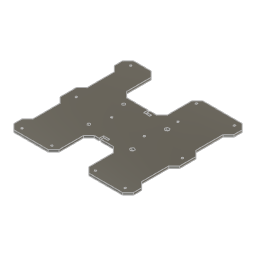
cr6_buildplate_carriage (Autodesk Fusion 360 design; units mm, degrees)
Autodesk Fusion 360 part; units mm, degrees
note: some values were not read from the file. Set by a fixed rule: the direction of a hole.
sketch "Sketch1" plane through (0, 0, 0) normal (0, 0, 1) x (1, 0, 0)
  line L0 (10, 0) -> (210, 0)
  line L1 (220, 10) -> (220, 210)
  line L2 (210, 220) -> (10, 220)
  line L3 (0, 210) -> (0, 10)
  line L4 (83, 0) -> (138, 0)
  line L5 (138, 0) -> (138, 55)
  line L6 (128, 65) -> (93, 65)
  line L7 (83, 55) -> (83, 0)
  line L8 (52.5, 220) -> (127.5, 220)
  line L9 (127.5, 220) -> (127.5, 165)
  line L10 (117.5, 155) -> (62.5, 155)
  line L11 (52.5, 165) -> (52.5, 220)
  line L12 (52.5, 165) -> (62.5, 155)
  line L13 (117.5, 155) -> (127.5, 165)
  line L14 (83, 55) -> (93, 65)
  line L15 (128, 65) -> (138, 55)
  line L16 (0, 25) -> (10, 25)
  line L17 (10, 25) -> (10, 95)
  line L18 (10, 95) -> (0, 95)
  line L19 (0, 95) -> (0, 25)
  line L20 (0, 125) -> (10, 125)
  line L21 (10, 125) -> (10, 195)
  line L22 (10, 195) -> (0, 195)
  line L23 (0, 195) -> (0, 125)
  line L24 (10, 220) -> (0, 210)
  line L25 (210, 220) -> (220, 210)
  line L26 (0, 10) -> (10, 0)
  line L27 (210, 0) -> (220, 10)
  line L28 (0, 95) -> (10, 85)
  line L29 (0, 125) -> (10, 135)
  line L30 (0, 195) -> (10, 185)
  line L31 (0, 25) -> (10, 35)
  line L32 (110, 0) -> (110, 220) construction
  line L33 (210, 195) -> (220, 195)
  line L34 (220, 195) -> (210, 185)
  line L35 (210, 125) -> (210, 195)
  line L36 (220, 125) -> (210, 135)
  line L37 (220, 125) -> (210, 125)
  line L38 (210, 95) -> (220, 95)
  line L39 (210, 25) -> (210, 95)
  line L40 (220, 95) -> (210, 85)
  line L41 (220, 25) -> (210, 25)
  line L42 (220, 25) -> (210, 35)
  line L43 (0, 110) -> (220, 110) construction
  line L44 (150, 142) -> (70, 142) construction
  line L45 (70, 142) -> (70, 78) construction
  line L46 (70, 78) -> (150, 78) construction
  line L47 (150, 78) -> (150, 142) construction
  line L48 (150, 142) -> (70, 78) construction
  line L49 (70, 142) -> (150, 78) construction
  line L50 (102, 65) -> (102, 73)
  line L51 (102, 73) -> (113, 73)
  line L52 (113, 73) -> (113, 70)
  line L53 (113, 70) -> (105, 70)
  line L54 (105, 70) -> (105, 65)
  line L55 (102, 155) -> (102, 147)
  line L56 (102, 147) -> (113, 147)
  line L57 (113, 150) -> (105, 150)
  line L58 (113, 147) -> (113, 150)
  line L59 (105, 150) -> (105, 155)
  line L60 (42.5, 220) -> (52.5, 210)
  line L61 (127.5, 210) -> (137.5, 220)
  line L62 (138, 10) -> (148, 0)
  line L63 (83, 10) -> (73, 0)
  point P0 (220, 0)
  point P1 (0, 220)
  point P2 (52.5, 155)
  point P3 (127.5, 155)
  point P4 (83, 65)
  point P5 (138, 65)
  point P6 (220, 220)
  point P7 (110, 110)
  point P8 (110, 110)
  dimension "d1" = 220
  dimension "d2" = 220
  dimension "d3" = 83
  dimension "d4" = 138
  dimension "d5" = 65
  dimension "d6" = 52.5
  dimension "d7" = 127.5
  dimension "d8" = 65
  dimension "d9" = 10
  dimension "d10" = 10
  dimension "d11" = 10
  dimension "d12" = 10
  dimension "d13" = 10
  dimension "d14" = 10
  dimension "d15" = 10
  dimension "d16" = 10
  dimension "d17" = 95
  dimension "d18" = 25
  dimension "d19" = 10
  dimension "d20" = 195
  dimension "d21" = 125
  dimension "d22" = 10
  dimension "d23" = 10
  dimension "d24" = 10
  dimension "d25" = 10
  dimension "d26" = 10
  dimension "d27" = 10
  dimension "d28" = 10
  dimension "d29" = 10
  dimension "d30" = 10
  dimension "d31" = 80
  dimension "d32" = 64
  dimension "d41" = 102
  dimension "d42" = 3
  dimension "d44" = 3
  dimension "d45" = 11
  dimension "d46" = 8
  dimension "d60" = 10
  dimension "d61" = 10
  dimension "d62" = 10
  dimension "d63" = 10
  constraint horizontal L0
  constraint vertical L1
  constraint horizontal L2
  constraint vertical L3
  constraint horizontal L4
  constraint vertical L5
  constraint horizontal L6
  constraint vertical L7
  constraint coincident L0 L4.start
  constraint horizontal L8
  constraint vertical L9
  constraint horizontal L10
  constraint vertical L11
  constraint coincident L2 L8.start
  constraint coincident L11 P2
  constraint coincident L10 P2
  constraint coincident L10 P3
  constraint coincident L9 P3
  constraint coincident L7 P4
  constraint coincident L6 P4
  constraint coincident L6 P5
  constraint coincident L5 P5
  constraint horizontal L16
  constraint vertical L17
  constraint horizontal L18
  constraint vertical L19
  constraint coincident L3 L16.start
  constraint horizontal L20
  constraint vertical L21
  constraint horizontal L22
  constraint vertical L23
  constraint coincident L3 L20.start
  constraint coincident P1 L2
  constraint coincident P1 L3
  constraint coincident L2 P6
  constraint coincident L1 P6
  constraint coincident origin L3
  constraint coincident origin L0
  constraint coincident P0 L0
  constraint coincident P0 L1
  constraint coincident L17 L28.end
  constraint coincident L21 L29.end
  constraint perpendicular L28 L29
  constraint coincident L21 L30.end
  constraint perpendicular L29 L30
  constraint coincident L17 L31.end
  constraint perpendicular L30 L31
  constraint midpoint L0 L32.start
  constraint midpoint L2 L32.end
  constraint symmetric L16.start L32 L41.start
  constraint symmetric L16.end L32 L39.start
  constraint symmetric L17.end L32 L38.start
  constraint symmetric L18.end L32 L38.end
  constraint symmetric L20.start L32 L36.start
  constraint symmetric L20.end L32 L35.start
  constraint symmetric L21.end L32 L33.start
  constraint symmetric L22.end L32 L33.end
  constraint symmetric L28.end L32 L40.end
  constraint symmetric L29.end L32 L36.end
  constraint symmetric L30.end L32 L34.end
  constraint symmetric L31.end L32 L42.end
  constraint midpoint L3 L43.start
  constraint midpoint L1 L43.end
  constraint midpoint L32 P8
  constraint horizontal L44
  constraint perpendicular L44 L45
  constraint parallel L44 L46
  constraint parallel L45 L47
  constraint coincident L48 P8
  constraint coincident L49 P8
  constraint coincident P8 P7
  constraint coincident L6 L50.start
  constraint perpendicular L6 L50
  constraint perpendicular L50 L51
  constraint perpendicular L51 L52
  constraint perpendicular L52 L53
  constraint coincident L6 L54.end
  constraint perpendicular L6 L54
  constraint symmetric L43 L50.start L55.start
  constraint symmetric L43 L50.end L55.end
  constraint symmetric L43 L51.end L56.end
  constraint symmetric L43 L52.end L57.start
  constraint symmetric L43 L53.end L57.end
  constraint symmetric L43 L54.end L59.end
  constraint coincident L2 L60.start
  constraint coincident L11 L60.end
  constraint perpendicular L24 L60
  constraint coincident L9 L61.start
  constraint coincident L2 L61.end
  constraint perpendicular L60 L61
  constraint coincident L5 L62.start
  constraint coincident L0 L62.end
  constraint perpendicular L61 L62
  constraint coincident L7 L63.start
  constraint coincident L0 L63.end
  constraint perpendicular L62 L63
  measures "d1" distance of origin P0
  measures "d2" distance of origin P1
  measures "d3" distance of L3 L7
  measures "d4" distance of L3 L5
  measures "d5" distance of L0 L6
  measures "d6" distance of L3 L11
  measures "d7" distance of L3 L9
  measures "d8" distance of L2 L10
  measures "d9" distance of L11.start P2
  measures "d10" distance of L10.end P2
  measures "d11" distance of L10.start P3
  measures "d12" distance of L9.end P3
  measures "d13" distance of L7.start P4
  measures "d14" distance of L6.end P4
  measures "d15" distance of L6.start P5
  measures "d16" distance of L5.end P5
  measures "d17" distance of L0 L18
  measures "d18" distance of L0 L16
  measures "d19" distance of L17 L19
  measures "d20" distance of L0 L22
  measures "d21" distance of L0 L20
  measures "d22" distance of L3 L21
  measures "d23" distance of P1 L2.end
  measures "d24" distance of P1 L3.start
  measures "d25" distance of L2.start P6
  measures "d26" distance of L1.end P6
  measures "d27" distance of origin L3.end
  measures "d28" distance of origin L0.start
  measures "d29" distance of P0 L0.end
  measures "d30" distance of P0 L1.start
  measures "d31" distance of L45.end L46.end
  measures "d32" distance of L44.end L45.end
  measures "d41" distance of L3 L50
  measures "d42" distance of L50 L54
  measures "d44" distance of L51 L53
  measures "d45" distance of L50 L52
  measures "d46" distance of L6 L51
  measures "d60" distance of L8.start L60.start
  measures "d61" distance of L8.end L61.end
  measures "d62" distance of L4.start L63.end
  measures "d63" horizontal distance of L62.start L62.end
extrude "Extrude1" add sketch "Sketch1" along normal blind 4 contours L0 L1 L2 L3 L5 L6 L7 L9 L10 L11 L12 L13 L14 L15 L16 L17 L18 L20 L21 L22 L24 L25 L26 L27 L33 L35 L37 L38 L39 L41 L50 L51 L52 L53 L54 L55 L56 L57 L58 L59 L60 L61 L62 L63 | L16 L17 L31 | L17 L18 L28 | L20 L21 L29 | L21 L22 L30 | L39 L41 L42 | L38 L39 L40 | L35 L36 L37 | L33 L34 L35
hole "Hole1" at (70, 142, 0) at (70, 78, 0) direction (0, 0, 1) diameter 5 end through all
hole "Hole2" at (150, 78, 0) at (150, 142, 0) direction (0, 0, 1) diameter 7.2 depth 4 tip angle 118
sketch "Sketch2" plane through (0, 0, 4) normal (0, 0, 1) x (-1, 0, 0)
  circle A0 centre (-150, -78) radius 3.6
  circle A1 centre (-150, -142) radius 3.6
  circle A2 centre (-70, -142) radius 2.5
  circle A3 centre (-70, -78) radius 2.5
  line L0 (-102, -155) -> (-62.5, -155)
  line L1 (-62.5, -155) -> (-52.5, -165)
  line L2 (-52.5, -165) -> (-52.5, -210)
  line L3 (-42.5, -220) -> (-10, -220)
  line L4 (-10, -220) -> (0, -210)
  line L5 (0, -210) -> (0, -195)
  line L6 (0, -195) -> (-10, -185)
  line L7 (-10, -185) -> (-10, -135)
  line L8 (-10, -135) -> (0, -125)
  line L9 (0, -125) -> (0, -95)
  line L10 (0, -95) -> (-10, -85)
  line L11 (-10, -85) -> (-10, -35)
  line L12 (-10, -35) -> (0, -25)
  line L13 (0, -25) -> (0, -10)
  line L14 (0, -10) -> (-10, 0)
  line L15 (-10, 0) -> (-73, 0)
  line L16 (-83, -10) -> (-83, -55)
  line L17 (-83, -55) -> (-93, -65)
  line L18 (-93, -65) -> (-102, -65)
  line L19 (-102, -65) -> (-102, -73)
  line L20 (-102, -73) -> (-113, -73)
  line L21 (-113, -73) -> (-113, -70)
  line L22 (-113, -70) -> (-105, -70)
  line L23 (-105, -70) -> (-105, -65)
  line L24 (-105, -65) -> (-128, -65)
  line L25 (-128, -65) -> (-138, -55)
  line L26 (-138, -55) -> (-138, -10)
  line L27 (-148, 0) -> (-210, 0)
  line L28 (-210, 0) -> (-220, -10)
  line L29 (-220, -10) -> (-220, -25)
  line L30 (-220, -25) -> (-210, -35)
  line L31 (-210, -35) -> (-210, -85)
  line L32 (-210, -85) -> (-220, -95)
  line L33 (-220, -95) -> (-220, -125)
  line L34 (-220, -125) -> (-210, -135)
  line L35 (-210, -135) -> (-210, -185)
  line L36 (-210, -185) -> (-220, -195)
  line L37 (-220, -195) -> (-220, -210)
  line L38 (-220, -210) -> (-210, -220)
  line L39 (-210, -220) -> (-137.5, -220)
  line L40 (-127.5, -210) -> (-127.5, -165)
  line L41 (-127.5, -165) -> (-117.5, -155)
  line L42 (-117.5, -155) -> (-105, -155)
  line L43 (-105, -155) -> (-105, -150)
  line L44 (-105, -150) -> (-113, -150)
  line L45 (-113, -150) -> (-113, -147)
  line L46 (-113, -147) -> (-102, -147)
  line L47 (-102, -147) -> (-102, -155)
  line L48 (0, -110) -> (-220, -110) construction
  line L49 (-10, 0) -> (-210, 0) construction
  line L50 (0, -10) -> (-220, -10) construction
  line L51 (0, -210) -> (-220, -210) construction
  line L52 (-138, -10) -> (-148, 0)
  line L53 (-137.5, -220) -> (-127.5, -210)
  line L54 (-52.5, -210) -> (-42.5, -220)
  line L55 (-73, 0) -> (-83, -10)
  point P0 (-15, -110)
  point P1 (-80, -110)
  point P2 (-140, -110)
  point P3 (-210, -110)
  point P4 (-15, -210)
  point P5 (-136, -210)
  point P6 (-206, -210)
  point P7 (-15, -10)
  point P8 (-70, -10)
  point P9 (-150, -10)
  point P10 (-205, -10)
  point P11 (-148, -164)
  dimension "d47" = 110
  dimension "d48" = 10
  dimension "d49" = 15
  dimension "d50" = 80
  dimension "d51" = 140
  dimension "d52" = 210
  dimension "d53" = 15
  dimension "d54" = 136
  dimension "d55" = 206
  dimension "d56" = 15
  dimension "d57" = 70
  dimension "d58" = 150
  dimension "d59" = 205
  dimension "d70" = 148
  dimension "d71" = 164
  constraint coincident L9 L48.start
  constraint coincident L33 L48.end
  constraint perpendicular L33 L48
  constraint coincident L13 L14.start
  constraint coincident L29 L28.end
  constraint perpendicular L29 L50
  constraint coincident L4.end L5.start
  constraint coincident L37.end L38.start
  constraint coincident L48 P0
  constraint coincident L48 P1
  constraint coincident L48 P2
  constraint coincident L48 P3
  constraint coincident L51 P4
  constraint coincident L51 P5
  constraint coincident L51 P6
  constraint coincident L50 P7
  constraint coincident L50 P8
  constraint coincident L50 P9
  constraint coincident L50 P10
  measures "d47" distance of L48 L49
  measures "d48" distance of L49 L50
  measures "d49" distance of L48.start P0
  measures "d50" distance of L48.start P1
  measures "d51" distance of L48.start P2
  measures "d52" distance of L48.start P3
  measures "d53" distance of L4.end P4
  measures "d54" distance of L4.end P5
  measures "d55" distance of L4.end P6
  measures "d56" distance of L13.end P7
  measures "d57" distance of L13.end P8
  measures "d58" distance of L13.end P9
  measures "d59" distance of L13.end P10
  measures "d70" distance of L9 P11
  measures "d71" distance of L27 P11
hole "Hole3" at (15, 210, 4) at (136, 210, 4) at (206, 210, 4) at (210, 110, 4) at (140, 110, 4) at (80, 110, 4) at (15, 110, 4) at (15, 10, 4) at (70, 10, 4) at (150, 10, 4) at (205, 10, 4) direction (0, 0, -1) diameter 3.332 depth 4 tip angle 118
thread "Thread1" "ANSI Metric M Profile 4.0 M4x0.7 6H"
hole "Hole5" at (148, 164, 4) direction (0, 0, -1) diameter 3.332 depth 4 tip angle 118
thread "Thread3" "ANSI Metric M Profile 4.0 M4x0.7 6H"
ref_plane "WorkPlane1" through (110, 110, 2) normal (-1, 0, 0) x (0, -1, 0)
equation "d10 = d9"
equation "d12 = d11"
equation "d14 = d13"
equation "d16 = d15"
equation "d24 = d23"
equation "d26 = d25"
equation "d28 = d27"
equation "d30 = d29"
